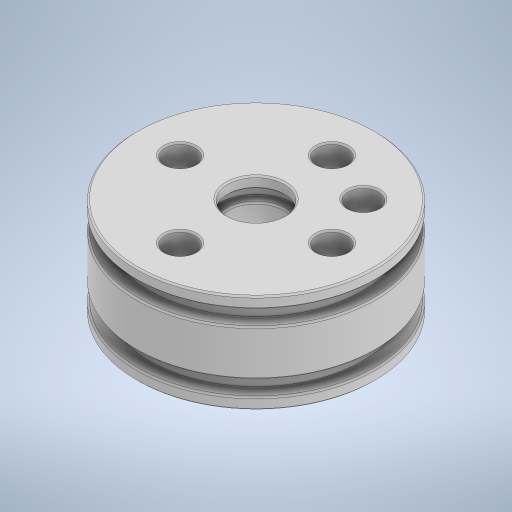
# Autodesk Inventor part: 2 Piston
Saved by Autodesk Inventor 2024 (Build 280153000, 153)
## iProperties
Created: 2024-04-17
Part Number: 2 Piston
Material: Generic
Document SubType Name: Modeling
Designer: Tommy Rohmann
Density: 1 g/cm^3
Appearance: Default
Author: Tommy Rohmann
Autodesk Inventor part; units mm, degrees
ref_plane "YZ Plane" through (0, 0, 0) normal (1, 0, 0) x (0, 1, 0)
ref_plane "XZ Plane" through (0, 0, 0) normal (0, 1, 0) x (-1, 0, 0)
ref_plane "XY Plane" through (0, 0, 0) normal (0, 0, 1) x (1, 0, 0)
sketch "Sketch1" plane through (0, 0, 0) normal (0, 0, 1) x (1, 0, 0)
  line L0 (50.8, 0) -> (50.8, 39.0312) construction
  line L1 (0, 0) -> (49.8475, 0)
  line L2 (44.45, 0) -> (44.45, 51.6727)
  line L3 (0, 0) -> (0, 50.5742)
  line L4 (49.8475, 0) -> (49.8475, 45.6895)
  line L5 (49.8475, 4.7625) -> (44.45, 4.7625)
  line L6 (44.45, 11.1125) -> (49.8475, 11.1125)
  line L7 (49.8475, 30.1625) -> (44.45, 30.1625)
  line L8 (44.45, 36.5125) -> (49.8475, 36.5125)
  line L9 (49.8475, 41.275) -> (0, 41.275)
  line L10 (11.8237, 0) -> (11.8237, 53.9909)
  line L11 (15.875, 0) -> (15.875, 48.05)
  line L12 (11.8237, 4.7625) -> (15.875, 4.7625)
  line L13 (15.875, 9.5377) -> (11.8237, 9.5377)
  line L14 (15.875, 31.7373) -> (11.8237, 31.7373)
  line L15 (11.8237, 36.5125) -> (15.875, 36.5125)
  point P0 (47.1487, 36.5125)
  point P1 (44.45, 30.1625)
  point P2 (11.8237, 41.275)
  dimension "d1" = 49.8475
  dimension "d2" = 44.45
  dimension "d3" = 6.35
  dimension "d4" = 6.35
  dimension "d5" = 4.7625
  dimension "d6" = 19.05
  dimension "d7" = 4.7625
  dimension "d12" = 41.275
  dimension "d20" = 11.8237
  dimension "d21" = 5.3975
  dimension "d22" = 15.875
  dimension "d23" = 4.7752
  dimension "d24" = 4.7752
  constraints: 32 end point, 20 point on line, 7 perpendicular, 4 vertical, 2 collinear, 2 horizontal, 1 midpoint
  measures "d1" distance of L1.start L1.end
  measures "d2" distance between parallel lines of L2 L3
  measures "d3" distance from line of point (47.149, 36.513) L7
  measures "d4" distance between parallel lines of L5 L6
  measures "d5" distance between parallel lines of L1 L5
  measures "d6" distance between parallel lines of L6 L7
  measures "d7" distance between parallel lines of L8 L9
  measures "d12" distance between parallel lines of L9 L1
  measures "d20" distance between parallel lines of L3 L10
  measures "d21" distance between parallel lines of L4 L2
  measures "d22" distance between parallel lines of L11 L3
  measures "d23" distance between parallel lines of L12 L13
  measures "d24" distance between parallel lines of L14 L15
revolve "Revolution1" add sketch "Sketch1" angle 360 about axis through (0, 0, 0) along (0, 1, 0) contours L10 L12 L11 L1 | L11 L9 L2 L1 | L9 L11 L15 L10 | L2 L5 L4 L1 | L10 L14 L11 L13 | L9 L4 L8 L2 | L2 L7 L4 L6
chamfer "Chamfer1" distance 0.635 angle 45 12 edges at (-49.8475, 0, 0) (-49.8475, 4.7625, 0) (-49.8475, 11.1125, 0) (-49.8475, 30.1625, 0) (-49.8475, 36.5125, 0) (-49.8475, 41.275, 0) (-11.8237, 41.275, 0) (-11.8237, 36.5125, 0) (-11.8237, 31.7373, 0) (-11.8237, 9.5377, 0) (-11.8237, 4.7625, 0) (-11.8237, 0, 0)
sketch "Sketch3" plane through (0, 41.275, 0) normal (0, 1, 0) x (1, 0, 0)
  circle A0 centre (0, 31.75) radius 6.35
  circle A1 centre (-31.75, 0) radius 6.35
  circle A2 centre (0, -31.75) radius 6.35
  circle A3 centre (31.75, 0) radius 6.35
  circle A4 centre (0, 0) radius 31.75 construction
  line L0 (0, 0) -> (22.4506, 22.4506) construction
  line L1 (0, 0) -> (31.75, 0) construction
  circle A5 centre (22.4506, 22.4506) radius 6.35
  dimension "d27" = 360
  dimension "d29" = 12.7
  dimension "d30" = 31.75
  dimension "d31" = 45
  dimension "d32" = 12.7
  constraints: 6 centre point, 4 end point, 2 coincident, 2 point on circle, 1 equal length, 1 horizontal, 9 other
  measures "d29" diameter of A0
  measures "d30" distance of A0.centre point (0, 0)
  measures "d31" angle of L1 L0
  measures "d32" diameter of A5
extrude "Extrusion3" cut sketch "Sketch3" against normal up to surface (30.1625 mm away) contours A0 | A1 | A2 | A3
extrude "Extrusion4" cut sketch "Sketch3" against normal blind 352.425 contours A5
chamfer "Chamfer2" distance 0.635 angle 45 5 edges at (-38.1, 41.275, 0) (-6.35, 41.275, -31.75) (16.1006, 41.275, -22.4506) (25.4, 41.275, 0) (-6.35, 41.275, 31.75)
body "Solid1"
